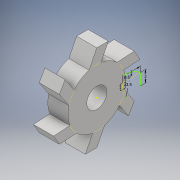
# Autodesk Inventor part: mtv_gear6_1-16
Saved by Autodesk Inventor 2018 (Build 220112000, 112)
## iProperties
Created: 2019-01-17
Part Number: mtv_gear6_1-16
Material: Generic
Document SubType Name: Modeling
Designer: aditya
Density: 1 g/cm^3
Appearance: Default
Author: aditya
## iProperties of the stored document mtv_gear6_1-16_3DPrint.ipt
Created: 2019-01-17
Part Number: mtv_gear6_1-16_3DPrint
Material: Generic
Document SubType Name: Modeling
Designer: aditya
Density: 1 g/cm^3
Appearance: Default
Author: aditya
Autodesk Inventor part; units mm, degrees
ref_plane "YZ Plane" through (0, 0, 0) normal (1, 0, 0) x (0, 1, 0)
ref_plane "XZ Plane" through (0, 0, 0) normal (0, 1, 0) x (-1, 0, 0)
ref_plane "XY Plane" through (0, 0, 0) normal (0, 0, 1) x (1, 0, 0)
sketch "Sketch1" plane through (0, 0, 0) normal (1, 0, 0) x (0, 1, 0)
  circle A0 centre (0, 0) radius 1.75
  circle A1 centre (0, 0) radius 5
  dimension "d0" = 3.5
  dimension "d1" = 10
  constraints: 2 centre point, 2 coincident
  measures "d0" diameter of A0
  measures "d1" diameter of A1
extrude "Extrusion1" add sketch "Sketch1" along normal blind 3.5
sketch "Sketch2" plane through (3.5, 0, 0) normal (1, 0, 0) x (0, 0, -1)
  circle A0 centre (0, 0) radius 5 construction
  line L0 (0, 5) -> (0, 4.5) construction
  line L1 (0, 4.5) -> (1, 4.5) construction
  line L2 (1, 4.5) -> (-1, 4.5) construction
  line L3 (0, 4.5) -> (0, 7.5) construction
  arc A1 (0, 7.5) -> (-1, 4.5) centre (2.4623, 5.0126) ccw
  line L4 (0, 7.5) -> (2, 7.5)
  dimension "d4" = 0.5
  dimension "d5" = 1
  dimension "d6" = 2
  dimension "d7" = 3
  dimension "d8" = 3.5
  dimension "d9" = 2
  constraints: 10 end point, 2 point on circle, 2 vertical, 1 centre point, 1 horizontal, 1 perpendicular, 1 point on line, 1 vertical alignment, 1 other
  measures "d4" distance of L0.start L0.end
  measures "d5" distance of L0.end L1.end
  measures "d6" distance of L1.end L2.end
  measures "d7" distance of L0.end L3.end
  measures "d8" radius of A1
  measures "d9" distance of L3.end L4.end
sketch "Sketch3" plane through (3.5, 0, 0) normal (1, 0, 0) x (0, 0, -1)
  circle A0 centre (0, 0) radius 5 construction
  line L0 (-5, 0) -> (-4.5, 0) construction
  line L1 (-4.5, 0) -> (-4.5, 1.5) construction
  line L2 (-4.5, 1.5) -> (-4.5, 0) construction
  line L3 (-4.5, 0) -> (-4.5, -1.5) construction
  line L4 (-5, 0) -> (-7.5, 0) construction
  line L5 (-7.5, 0) -> (-4.5, -1.5)
  line L6 (-7.5, 0) -> (-7.5, 2)
  line L7 (-7.5, 2) -> (-4.9474, 0.7237)
  line L8 (-4.5, -1.5) -> (-4.5, 0.5)
  line L9 (-4.9474, 0.7237) -> (-4.5, 0.5)
  dimension "d10" = 0.5
  dimension "d11" = 1.5
  dimension "d12" = 1.5
  dimension "d13" = 1.5
  dimension "d14" = 2.5
  dimension "d15" = 2
  constraints: 20 end point, 3 point on line, 2 horizontal, 2 perpendicular, 2 point on circle, 1 parallel, 1 vertical
  measures "d10" distance of L0.start L0.end
  measures "d11" distance of L0.end L1.end
  measures "d12" distance of L1.end L0.end
  measures "d13" distance of L0.end L3.end
  measures "d14" distance of L0.start L4.end
  measures "d15" distance of L4.end L6.end
extrude "Extrusion2" add sketch "Sketch3" against normal blind 3.5
pattern_circular "Circular Pattern1" count 6 over 360 about axis through (0, 0, 0) along (1, 0, 0) of "Extrusion2"
body "Solid1"
